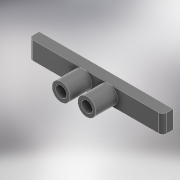
# Autodesk Inventor part: 6
Saved by Autodesk Inventor 2022 (Build 260153000, 153)
## iProperties
Created: 2023-12-25
Part Number: 6
Material: Generisch
Document SubType Name: Modeling
Designer: alsaa
Density: 1 g/cm^3
Appearance: Glatt - Schwarz
Author: alsaa
## iProperties of the stored document 6_3D-Druck.ipt
Created: 2023-12-25
Part Number: 6_3D-Druck
Material: Generisch
Document SubType Name: Modeling
Designer: alsaa
Density: 1 g/cm^3
Appearance: Vorgabe
Author: alsaa
Autodesk Inventor part; units mm, degrees
ref_plane "YZ Plane" through (0, 0, 0) normal (1, 0, 0) x (0, 1, 0)
ref_plane "XZ Plane" through (0, 0, 0) normal (0, 1, 0) x (-1, 0, 0)
ref_plane "XY Plane" through (0, 0, 0) normal (0, 0, 1) x (1, 0, 0)
sketch "Skizze1" plane through (0, 0, 0) normal (0, 0, 1) x (1, 0, 0)
  circle A0 centre (-5, 0) radius 2.15
  circle A1 centre (-5, 0) radius 3.5
  line L0 (-15.4774, 0) -> (15.4774, 0) construction
  line L1 (0, 6.6843) -> (0, -6.6843) construction
  circle A2 centre (5, 0) radius 2.15
  circle A3 centre (5, 0) radius 3.5
  line L2 (-8.5, 3.5) -> (8.5, 3.5)
  line L3 (8.5, 3.5) -> (8.5, -3.5)
  line L4 (8.5, -3.5) -> (-8.5, -3.5)
  line L5 (-8.5, -3.5) -> (-8.5, 3.5)
  line L6 (26, -3.5) -> (-26, -3.5)
  line L7 (-26, -3.5) -> (-26, 3.5)
  line L8 (-26, 3.5) -> (26, 3.5)
  line L9 (26, 3.5) -> (26, -3.5)
  line L10 (26, -3.5) -> (-26, 3.5) construction
  line L11 (-26, -3.5) -> (26, 3.5) construction
  point P0 (0, 0)
  point P1 (0, 0)
  dimension "d0" = 4.3
  dimension "d1" = 7
  dimension "d2" = 10
  dimension "d7" = 52
  constraints: 24 end point, 4 centre point, 4 midpoint, 4 parallel, 4 tangent, 3 coincident, 3 horizontal, 2 perpendicular, 2 point on line, 2 symmetric about line, 1 vertical, 2 other
  measures "d0" diameter of A0
  measures "d1" diameter of A1
  measures "d2" distance of A2.centre A0.centre
  measures "d7" distance of L7.end L8.end
extrude "Extrusion1" add sketch "Skizze1" along normal blind 12.5 contours A1 | A3
extrude "Extrusion2" add sketch "Skizze1" along normal blind 4
chamfer "Fase1" [suppressed]
fillet "Rundung1" radius 1.5 2 edges at (-26, 0, 4) (26, 0, 4)
